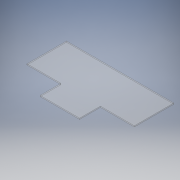
# Autodesk Inventor part: Electronics Plate
Saved by Autodesk Inventor 2017 (Build 210142000, 142)
## iProperties
Created: 2017-01-20
Part Number: Electronics Plate
Material: Generic
Document SubType Name: Modeling
Designer: Ben
Density: 1 g/cm^3
Appearance: Polycarbonate - Clear
Author: Ben
Autodesk Inventor part; units mm, degrees
ref_plane "YZ Plane" through (0, 0, 0) normal (1, 0, 0) x (0, 1, 0)
ref_plane "XZ Plane" through (0, 0, 0) normal (0, 1, 0) x (-1, 0, 0)
ref_plane "XY Plane" through (0, 0, 0) normal (0, 0, 1) x (1, 0, 0)
sketch "Sketch1" plane through (0, 0, 0) normal (0, 1, 0) x (-1, 0, 0)
  line L0 (311.15, -349.25) -> (-311.15, -349.25)
  line L1 (-311.15, -349.25) -> (-311.15, -120.65)
  line L2 (311.15, -120.65) -> (311.15, -349.25)
  line L3 (311.15, -120.65) -> (114.3, -120.65)
  line L4 (114.3, -120.65) -> (114.3, 0)
  line L5 (114.3, 0) -> (-114.3, 0)
  line L6 (-114.3, 0) -> (-114.3, -120.65)
  line L7 (-114.3, -120.65) -> (-311.15, -120.65)
  point P0 (0, 0)
  point P1 (0, 0)
  point P2 (0, 0)
  dimension "d0" = 228.6
  dimension "d1" = 622.3
  dimension "d2" = 228.6
  dimension "d3" = 349.25
  constraints: 16 end point, 5 perpendicular, 2 coincident, 2 equal length, 2 horizontal, 1 midpoint, 1 parallel, 1 point on line
  measures "d0" distance of L2.start L0.start
  measures "d1" distance of L0.start L0.end
  measures "d2" distance of L4.end L5.end
  measures "d3" distance between parallel lines of L5 L0
extrude "Extrusion1" add sketch "Sketch1" along normal blind 6.35
body "Solid1"
